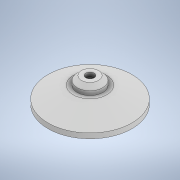
# Autodesk Inventor part: driven gear addon
Saved by Autodesk Inventor 2022 (Build 260153000, 153)
## iProperties
Created: 2021-11-13
Part Number: driven gear addon
Material: Generic
Document SubType Name: Modeling
Designer: a-dubs
Density: 1 g/cm^3
Appearance: Default
Author: a-dubs
Autodesk Inventor part; units mm, degrees
ref_plane "YZ Plane" through (0, 0, 0) normal (1, 0, 0) x (0, 1, 0)
ref_plane "XZ Plane" through (0, 0, 0) normal (0, 1, 0) x (-1, 0, 0)
ref_plane "XY Plane" through (0, 0, 0) normal (0, 0, 1) x (1, 0, 0)
sketch "Sketch1" plane through (0, 0, 0) normal (0, 1, 0) x (-1, 0, 0)
  circle A0 centre (0, 0) radius 6.125
  line L0 (0, 6.125) -> (0, 9.125)
  circle A1 centre (0, 0) radius 9.125
  line L1 (0, 0) -> (30, 0)
  circle A2 centre (0, 0) radius 30
  circle A3 centre (0, 0) radius 3
  dimension "d0" = 12.25
  dimension "d1" = 3
  dimension "d2" = 30
  dimension "d10" = 6
  constraints: 4 coincident, 4 end point, 2 vertical alignment, 1 centre point, 1 horizontal, 1 horizontal alignment, 1 vertical, 6 other
  measures "d1" distance of L0.start L0.end
  measures "d2" distance of L1.start L1.end
  measures "d10" diameter of A3
extrude "Extrusion1" add sketch "Sketch1" along normal blind 12 contours L1 A1 L0 A0 | A0 L0 A1 L1 | A2
chamfer "Chamfer2" distance 18 angle 25 1 edges at (30, 12, 0) measured on face at (29.5, 12, 0)
extrude "Extrusion3" add sketch "Sketch1" along normal blind 6 from surface at 12 contours A0 | L1 A1 L0 A0 | A0 L0 A1 L1
chamfer "Chamfer3" distance 3 angle 45 1 edges at (9.125, 18, 0)
chamfer "Chamfer4" distance 3.1 angle 45 1 edges at (3, 12, 0)
body "Solid1"
